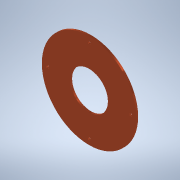
# Autodesk Inventor part: second copper plate
Saved by Autodesk Inventor 2020 (Build 240168000, 168)
## iProperties
Created: 2021-01-05
Part Number: second copper plate
Material: Copper
Document SubType Name: Modeling
Designer: Vikki
Density: 8.94 g/cm^3
Appearance: Copper - Satin
Mass: 2097.45 g
Surface Area: 990.607 cm^2
Volume: 234.614 cm^3
Author: Vikki
Autodesk Inventor part; units mm, degrees
ref_plane "YZ Plane" through (0, 0, 0) normal (1, 0, 0) x (0, 1, 0)
ref_plane "XZ Plane" through (0, 0, 0) normal (0, 1, 0) x (-1, 0, 0)
ref_plane "XY Plane" through (0, 0, 0) normal (0, 0, 1) x (1, 0, 0)
sketch "Sketch1" plane through (0, 0, 0) normal (0, 0, 1) x (1, 0, 0)
  circle A0 centre (0, -110) radius 125 projected
  circle A1 centre (0, -220) radius 4 projected
  circle A2 centre (110, -110) radius 4 projected
  circle A3 centre (-110, -110) radius 4 projected
  circle A4 centre (0, 0) radius 4 projected
  circle A5 centre (0, -110) radius 125 projected
  circle A6 centre (-7.5, -97.0096) radius 2 construction
  circle A7 centre (-15, -110) radius 2 construction
  circle A8 centre (-7.5, -122.9904) radius 2 construction
  circle A9 centre (7.5, -122.9904) radius 2 construction
  circle A10 centre (15, -110) radius 2 construction
  circle A11 centre (7.5, -97.0096) radius 2 construction
  circle A12 centre (0, -110) radius 29
  dimension "d0" = 58
  constraints: 1 centre point, 1 coincident
  measures "d0" diameter of A12
extrude "Extrusion1" add sketch "Sketch1" along normal blind 5
body "Solid1"
